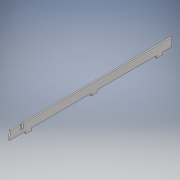
# Autodesk Inventor part: wall outer plunger
Saved by Autodesk Inventor 2017 (Build 210142000, 142)
## iProperties
Created: 2017-02-21
Part Number: wall outer plunger
Material: Generic
Document SubType Name: Modeling
Designer: John
Density: 1 g/cm^3
Appearance: Default
Author: John
Autodesk Inventor part; units mm, degrees
ref_plane "YZ Plane" through (0, 0, 0) normal (1, 0, 0) x (0, 1, 0)
ref_plane "XZ Plane" through (0, 0, 0) normal (0, 1, 0) x (-1, 0, 0)
ref_plane "XY Plane" through (0, 0, 0) normal (0, 0, 1) x (1, 0, 0)
sketch "Sketch2" plane through (0, 0, 0) normal (0, 1, 0) x (-1, 0, 0)
  line L0 (-1.5, -198.6195) -> (1.5, -198.6195)
  line L1 (1.5, -198.6195) -> (1.5, 198.6195)
  line L2 (1.5, 198.6195) -> (-1.5, 198.6195)
  line L3 (-1.5, 198.6195) -> (-1.5, -198.6195)
  line L4 (-1.5, -198.6195) -> (1.5, 198.6195) construction
  line L5 (1.5, -198.6195) -> (-1.5, 198.6195) construction
  point P0 (0, 0)
  dimension "d0" = 3
  dimension "d1" = 397.239
  constraints: 12 end point, 2 midpoint, 2 parallel, 1 horizontal, 1 perpendicular
  measures "d0" distance of L2.end L1.end
  measures "d1" distance of L1.end L0.end
extrude "Extrusion1" add sketch "Sketch2" along normal blind 20
sketch "Sketch4" plane through (1.5, 0, -198.6195) normal (1, 0, 0) x (0, 0, -1)
  line L0 (0, 0) -> (-397.239, 0) projected
  line L1 (-397.239, 0) -> (-397.239, 20) projected
  line L2 (-397.239, 0) -> (-397.239, 20)
  line L3 (-397.239, 20) -> (-393.7125, 20)
  line L4 (-397.239, 20) -> (0, 20) projected
  line L5 (-397.239, 0) -> (-393.7125, 20)
  point P0 (-198.6195, 0)
  point P1 (-329.239, 0)
  dimension "d10" = 10
  constraints: 6 end point, 1 point on line, 1 vertical
  measures "d10" angle of L1 L5
extrude "Extrusion3" cut sketch "Sketch4" against normal through all
sketch "Sketch6" plane through (1.5, 0, -198.6195) normal (1, 0, 0) x (0, 0, -1)
  line L0 (-393.7125, 20) -> (0, 20) projected
  line L1 (-369.839, 20) -> (-363.839, 20)
  line L2 (-363.839, 20) -> (-363.839, 8)
  line L3 (-363.839, 8) -> (-369.839, 8)
  line L4 (-369.839, 8) -> (-369.839, 20)
  line L5 (-397.239, 0) -> (0, 0) construction
  line L6 (-397.239, 0) -> (-397.239, 30) construction
  point P0 (-198.6195, 0)
  dimension "d20" = 6
  dimension "d21" = 12
  dimension "d25" = 27.4
  constraints: 10 end point, 2 parallel, 1 horizontal, 1 perpendicular, 1 point on line, 1 vertical
  measures "d20" distance of L2.end L3.end
  measures "d21" distance of L1.end L2.end
  measures "d25" distance between parallel lines of L4 L6
extrude "Extrusion5" cut sketch "Sketch6" against normal blind 6
sketch "Sketch7" plane through (1.5, 0, -198.6195) normal (1, 0, 0) x (0, 0, -1)
  line L0 (0, 0) -> (-397.239, 0) projected
  line L1 (-357.239, 0) -> (-342.239, 0)
  line L2 (-342.239, 0) -> (-342.239, -6)
  line L3 (-342.239, -6) -> (-357.239, -6)
  line L4 (-357.239, -6) -> (-357.239, 0)
  line L5 (-197.239, 0) -> (-182.239, 0)
  line L6 (-182.239, 0) -> (-182.239, -6)
  line L7 (-182.239, -6) -> (-197.239, -6)
  line L8 (-197.239, -6) -> (-197.239, 0)
  line L9 (-37.239, 0) -> (-22.239, 0)
  line L10 (-22.239, 0) -> (-22.239, -6)
  line L11 (-22.239, -6) -> (-37.239, -6)
  line L12 (-37.239, -6) -> (-37.239, 0)
  point P0 (-198.6195, 0)
  dimension "d26" = 15
  dimension "d27" = 6
  dimension "d28" = 15
  dimension "d29" = 15
  dimension "d30" = 6
  dimension "d31" = 40
  dimension "d32" = 145
  dimension "d33" = 145
  constraints: 24 end point, 6 parallel, 3 horizontal, 3 perpendicular, 2 collinear, 1 point on line
  measures "d26" distance of L2.end L3.end
  measures "d27" distance of L1.end L2.end
  measures "d28" distance of L6.end L7.end
  measures "d29" distance of L10.end L11.end
  measures "d30" distance of L9.end L10.end
  measures "d31" distance from line of L4 L0.end
  measures "d32" distance between parallel lines of L12 L6
  measures "d33" distance between parallel lines of L2 L8
extrude "Extrusion6" add sketch "Sketch7" against normal blind 3
body "Solid1"
